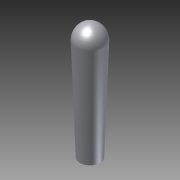
# Autodesk Inventor part: AA-toggle-toggle
Saved by Autodesk Inventor 2011 SP1 (Build 150282100, 282)
## iProperties
Created: 2013-12-24
Part Number: AA-toggle-toggle
Catalog Web Link: www.cadenas.de
Description: A Series - Process Sealed Subminiature Toggle - toggle-
Vendor: NKKSWITCHES
Document SubType Name: Modeling
Designer: PARTuser1
Manufacturer: NKKSWITCHES
Density: 1 g/cm^3
Category: PARTsolutions
Company: NKKSWITCHES
Title: AA-toggle-toggle
Author: Cadenas PARTsolutions
PSOL_IDENT_0: {$CADENAS_DATA\23d-libs\nkkswitches\toggle\a\parts\a_toggle_toggle.prj},227 {VTYP=3D},{NB=AA-toggle-
PSOL_IDENT_1: toggle},{LINA=AA-toggle-toggle},{NN=A Series - Process Sealed Subminiature Toggle - toggle},{DATE=12
PSOL_IDENT_2: .03.2009 11:54:50},{GEOMDATE=12.03.2009 00:00:00},{VERSION=},{LINEID=10},{LINESUBID=-1},{WBVAR=TGGLS
PSOL_IDENT_3: }  {NB=AA-toggle-toggle},{LINA=AA-toggle-toggle},{KT=DUMMY},{PN=AA},{SRS=A},{TGGLS=A},{TGGLSCLR=0.95
PSOL_IDENT_4: ,0.95,0.95,0.00}
CNS_NN: A Series - Process Sealed Subminiature Toggle - toggle
CNS_NB: AA-toggle-toggle
CNS_NBSYN: $PN.-toggle-toggle
CNS_LINA: AA-toggle-toggle
CNS_PN: AA
CNS_SRS: A
CNS_TGGLS: A - .394 (10.0mm) Bat
CNS_TGGLSCLR: 0.95,0.95,0.95,0.00
SUPPLIER: NKKSWITCHES
ARTICLENO: AA-toggle-toggle
BOMINFO: AA-toggle-toggle
CREATOR: CADENAS GmbH
Autodesk Inventor part; units mm, degrees
sketch "Sketch_1" plane through (0, 0, 0) normal (1, 0, 0) x (0, 1, 0)
  line L0 (10.0076, 0) -> (-1.016, 0)
  line L1 (-1.016, 0) -> (-1.016, 0.9592)
  line L2 (-1.016, 0.9592) -> (8.6106, 1.2954)
  arc A0 (10.0076, 0) -> (8.6106, 1.2954) centre (8.6143, -0.1016) ccw
  line L3 (10.0076, 0) -> (-1.016, 0)
  constraints: 8 end point, 2 point on circle, 1 centre point
revolve "Revolution1" add sketch "Sketch_1" angle 360 about axis through (0, 10.0076, 0) along (0, 1, 0)
ref_plane "to_body1_XY" through (0, 0, 0) normal (0, 1, 0) x (1, 0, 0)
ref_plane "to_body1_YZ" through (0, 0, 0) normal (1, 0, 0) x (0, 0, -1)
ref_plane "to_body1_ZX" through (0, 0, 0) normal (0, 0, -1) x (0, 1, 0)
body "Solid1"
